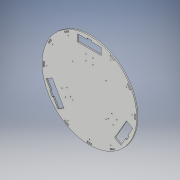
# Autodesk Inventor part: De_final
Saved by Autodesk Inventor 2019 (Build 230136000, 136)
## iProperties
Created: 2021-01-20
Part Number: De_final
Material: Generic
Document SubType Name: Modeling
Designer: Admin
Density: 1 g/cm^3
Appearance: Default
Author: Admin
Autodesk Inventor part; units mm, degrees
ref_plane "YZ Plane" through (0, 0, 0) normal (1, 0, 0) x (0, 1, 0)
ref_plane "XZ Plane" through (0, 0, 0) normal (0, 1, 0) x (-1, 0, 0)
ref_plane "XY Plane" through (0, 0, 0) normal (0, 0, 1) x (1, 0, 0)
sketch "Sketch1" plane through (0, 0, 0) normal (0, 0, 1) x (1, 0, 0)
  circle A0 centre (-100.7807, -75.4427) radius 1.73
  circle A1 centre (-79.9441, -63.4127) radius 1.73
  circle A2 centre (79.9441, -63.4127) radius 1.73
  circle A3 centre (115.7257, -49.5573) radius 1.73
  circle A4 centre (94.8891, -37.5273) radius 1.73
  circle A5 centre (100.7807, -75.4427) radius 1.73
  circle A6 centre (-14.945, 125) radius 1.73
  circle A7 centre (-14.945, 100.94) radius 1.73
  circle A8 centre (14.945, 125) radius 1.73
  line L0 (10, 182.5) -> (10, 187.5)
  line L1 (10, 187.5) -> (0, 187.5)
  line L2 (50, 182.5) -> (10, 182.5)
  circle A9 centre (-94.8891, -37.5273) radius 1.73
  circle A10 centre (-115.7257, -49.5573) radius 1.73
  circle A11 centre (0, 0) radius 200
  circle A12 centre (14.945, 100.94) radius 1.73
  line L3 (0, 152.5) -> (50, 152.5)
  line L4 (50, 152.5) -> (50, 182.5)
  line L5 (0, 152.5) -> (-50, 152.5)
  line L6 (-10, 187.5) -> (0, 187.5)
  line L7 (-10, 182.5) -> (-10, 187.5)
  line L8 (-50, 182.5) -> (-10, 182.5)
  line L9 (-50, 152.5) -> (-50, 182.5)
  circle A13 centre (0, 0) radius 200
  line L10 (-163.0496, -82.5897) -> (-167.3798, -85.0897)
  line L11 (-167.3798, -85.0897) -> (-162.3798, -93.75)
  line L12 (-183.0496, -47.9487) -> (-163.0496, -82.5897)
  line L13 (-132.0689, -76.25) -> (-157.0689, -32.9487)
  line L14 (-157.0689, -32.9487) -> (-183.0496, -47.9487)
  line L15 (-132.0689, -76.25) -> (-107.0689, -119.5513)
  line L16 (-157.3798, -102.4103) -> (-162.3798, -93.75)
  line L17 (-153.0496, -99.9103) -> (-157.3798, -102.4103)
  line L18 (-133.0496, -134.5513) -> (-153.0496, -99.9103)
  line L19 (-107.0689, -119.5513) -> (-133.0496, -134.5513)
  circle A14 centre (0, 0) radius 200
  line L20 (153.0496, -99.9103) -> (157.3798, -102.4103)
  line L21 (157.3798, -102.4103) -> (162.3798, -93.75)
  line L22 (133.0496, -134.5513) -> (153.0496, -99.9103)
  line L23 (132.0689, -76.25) -> (107.0689, -119.5513)
  line L24 (107.0689, -119.5513) -> (133.0496, -134.5513)
  line L25 (132.0689, -76.25) -> (157.0689, -32.9487)
  line L26 (167.3798, -85.0897) -> (162.3798, -93.75)
  line L27 (163.0496, -82.5897) -> (167.3798, -85.0897)
  line L28 (183.0496, -47.9487) -> (163.0496, -82.5897)
  line L29 (157.0689, -32.9487) -> (183.0496, -47.9487)
  dimension "d4" = 40
  dimension "d5" = 3.46
  dimension "d6" = 360
  dimension "d7" = 50
  dimension "d8" = 360
  constraints: 60 end point, 15 centre point, 2 coincident, 2 perpendicular, 1 horizontal, 90 other
  measures "d4" distance of L2.start L0.start
  measures "d5" diameter of A8
  measures "d7" distance of L3.start L3.end
extrude "Extrusion1" add sketch "Sketch1" along normal blind 5
sketch "Sketch2" plane through (0, 0, 5) normal (0, 0, 1) x (1, 0, 0)
  circle A0 centre (0, 0) radius 195 construction
  line L0 (0, 195) -> (10, 195)
  line L1 (10, 195) -> (10, 190)
  line L2 (10, 190) -> (0, 190)
  circle A1 centre (0, 0) radius 195 construction
  line L3 (0, 195) -> (-10, 195)
  line L4 (-10, 195) -> (-10, 190)
  line L5 (-10, 190) -> (0, 190)
  circle A2 centre (0, 0) radius 195 construction
  line L6 (97.5, 168.875) -> (106.1603, 163.875)
  line L7 (106.1603, 163.875) -> (103.6603, 159.5448)
  line L8 (103.6603, 159.5448) -> (95, 164.5448)
  circle A3 centre (0, 0) radius 195 construction
  line L9 (97.5, 168.875) -> (88.8397, 173.875)
  line L10 (88.8397, 173.875) -> (86.3397, 169.5448)
  line L11 (86.3397, 169.5448) -> (95, 164.5448)
  circle A4 centre (0, 0) radius 195 construction
  line L12 (168.875, 97.5) -> (173.875, 88.8397)
  line L13 (173.875, 88.8397) -> (169.5448, 86.3397)
  line L14 (169.5448, 86.3397) -> (164.5448, 95)
  circle A5 centre (0, 0) radius 195 construction
  line L15 (168.875, 97.5) -> (163.875, 106.1603)
  line L16 (163.875, 106.1603) -> (159.5448, 103.6603)
  line L17 (159.5448, 103.6603) -> (164.5448, 95)
  circle A6 centre (0, 0) radius 195 construction
  line L18 (195, 0) -> (195, -10)
  line L19 (195, -10) -> (190, -10)
  line L20 (190, -10) -> (190, 0)
  circle A7 centre (0, 0) radius 195 construction
  line L21 (195, 0) -> (195, 10)
  line L22 (195, 10) -> (190, 10)
  line L23 (190, 10) -> (190, 0)
  circle A8 centre (0, 0) radius 195 construction
  line L24 (168.875, -97.5) -> (163.875, -106.1603)
  line L25 (163.875, -106.1603) -> (159.5448, -103.6603)
  line L26 (159.5448, -103.6603) -> (164.5448, -95)
  circle A9 centre (0, 0) radius 195 construction
  line L27 (168.875, -97.5) -> (173.875, -88.8397)
  line L28 (173.875, -88.8397) -> (169.5448, -86.3397)
  line L29 (169.5448, -86.3397) -> (164.5448, -95)
  circle A10 centre (0, 0) radius 195 construction
  line L30 (97.5, -168.875) -> (88.8397, -173.875)
  line L31 (88.8397, -173.875) -> (86.3397, -169.5448)
  line L32 (86.3397, -169.5448) -> (95, -164.5448)
  circle A11 centre (0, 0) radius 195 construction
  line L33 (97.5, -168.875) -> (106.1603, -163.875)
  line L34 (106.1603, -163.875) -> (103.6603, -159.5448)
  line L35 (103.6603, -159.5448) -> (95, -164.5448)
  circle A12 centre (0, 0) radius 195 construction
  line L36 (0, -195) -> (-10, -195)
  line L37 (-10, -195) -> (-10, -190)
  line L38 (-10, -190) -> (0, -190)
  circle A13 centre (0, 0) radius 195 construction
  line L39 (0, -195) -> (10, -195)
  line L40 (10, -195) -> (10, -190)
  line L41 (10, -190) -> (0, -190)
  circle A14 centre (0, 0) radius 195 construction
  line L42 (-97.5, -168.875) -> (-106.1603, -163.875)
  line L43 (-106.1603, -163.875) -> (-103.6603, -159.5448)
  line L44 (-103.6603, -159.5448) -> (-95, -164.5448)
  circle A15 centre (0, 0) radius 195 construction
  line L45 (-97.5, -168.875) -> (-88.8397, -173.875)
  line L46 (-88.8397, -173.875) -> (-86.3397, -169.5448)
  line L47 (-86.3397, -169.5448) -> (-95, -164.5448)
  circle A16 centre (0, 0) radius 195 construction
  line L48 (-168.875, -97.5) -> (-173.875, -88.8397)
  line L49 (-173.875, -88.8397) -> (-169.5448, -86.3397)
  line L50 (-169.5448, -86.3397) -> (-164.5448, -95)
  circle A17 centre (0, 0) radius 195 construction
  line L51 (-168.875, -97.5) -> (-163.875, -106.1603)
  line L52 (-163.875, -106.1603) -> (-159.5448, -103.6603)
  line L53 (-159.5448, -103.6603) -> (-164.5448, -95)
  circle A18 centre (0, 0) radius 195 construction
  line L54 (-195, 0) -> (-195, 10)
  line L55 (-195, 10) -> (-190, 10)
  line L56 (-190, 10) -> (-190, 0)
  circle A19 centre (0, 0) radius 195 construction
  line L57 (-195, 0) -> (-195, -10)
  line L58 (-195, -10) -> (-190, -10)
  line L59 (-190, -10) -> (-190, 0)
  circle A20 centre (0, 0) radius 195 construction
  line L60 (-168.875, 97.5) -> (-163.875, 106.1603)
  line L61 (-163.875, 106.1603) -> (-159.5448, 103.6603)
  line L62 (-159.5448, 103.6603) -> (-164.5448, 95)
  circle A21 centre (0, 0) radius 195 construction
  line L63 (-168.875, 97.5) -> (-173.875, 88.8397)
  line L64 (-173.875, 88.8397) -> (-169.5448, 86.3397)
  line L65 (-169.5448, 86.3397) -> (-164.5448, 95)
  circle A22 centre (0, 0) radius 195 construction
  line L66 (-97.5, 168.875) -> (-88.8397, 173.875)
  line L67 (-88.8397, 173.875) -> (-86.3397, 169.5448)
  line L68 (-86.3397, 169.5448) -> (-95, 164.5448)
  circle A23 centre (0, 0) radius 195 construction
  line L69 (-97.5, 168.875) -> (-106.1603, 163.875)
  line L70 (-106.1603, 163.875) -> (-103.6603, 159.5448)
  line L71 (-103.6603, 159.5448) -> (-95, 164.5448)
  dimension "d11" = 390
  dimension "d12" = 10
  dimension "d13" = 5
  dimension "d16" = 360
  constraints: 144 end point, 4 horizontal alignment, 4 vertical alignment, 3 coincident, 1 horizontal, 1 parallel, 1 perpendicular, 242 other
  measures "d12" distance of L1.end L2.end
  measures "d13" distance of L0.end L1.end
extrude "Extrusion2" cut sketch "Sketch2" against normal blind 5 contours L6 L7 L8 L11 L10 L9 | L12 L13 L14 L17 L16 L15 | L18 L19 L20 L23 L22 L21 | L30 L31 L32 L35 L34 L33 | L36 L37 L38 L41 L40 L39 | L42 L43 L44 L47 L46 L45 | L54 L55 L56 L59 L58 L57 | L60 L61 L62 L65 L64 L63 | L66 L67 L68 L71 L70 L69
sketch "Sketch3" plane through (0, 0, 5) normal (0, 0, 1) x (1, 0, 0)
  line L0 (88.8397, 173.875) -> (106.1603, 163.875) projected
  circle A0 centre (90, 155.8846) radius 1.5
  circle A1 centre (0, 180) radius 1.5
  circle A2 centre (-90, 155.8846) radius 1.5
  circle A3 centre (-155.8846, 90) radius 1.5
  circle A4 centre (-180, 0) radius 1.5
  circle A5 centre (-155.8846, -90) radius 1.5
  circle A6 centre (-90, -155.8846) radius 1.5
  circle A7 centre (0, -180) radius 1.5
  circle A8 centre (90, -155.8846) radius 1.5
  circle A9 centre (155.8846, -90) radius 1.5
  circle A10 centre (180, 0) radius 1.5
  circle A11 centre (155.8846, 90) radius 1.5
  point P0 (0, 0)
  point P1 (0, 0)
  dimension "d21" = 3
  dimension "d24" = 360
  constraints: 12 centre point, 1 coincident, 25 other
  measures "d21" diameter of A0
extrude "Extrusion3" cut sketch "Sketch3" against normal blind 5 contours A0 | A2 | A3 | A4 | A6 | A7 | A8 | A10 | A11
sketch "Sketch4" plane through (0, 0, 5) normal (0, 0, 1) x (1, 0, 0)
  line L0 (0, 0) -> (100, 0) construction
  circle A0 centre (70.7107, 70.7107) radius 1.5
  circle A1 centre (-70.7107, 70.7107) radius 1.5
  circle A2 centre (-70.7107, -70.7107) radius 1.5
  circle A3 centre (70.7107, -70.7107) radius 1.5
  dimension "d30" = 3
  dimension "d33" = 360
  constraints: 4 centre point, 2 end point, 1 coincident, 1 horizontal, 9 other
  measures "d30" diameter of A0
extrude "Extrusion4" cut sketch "Sketch4" against normal blind 5
body "Solid1"
